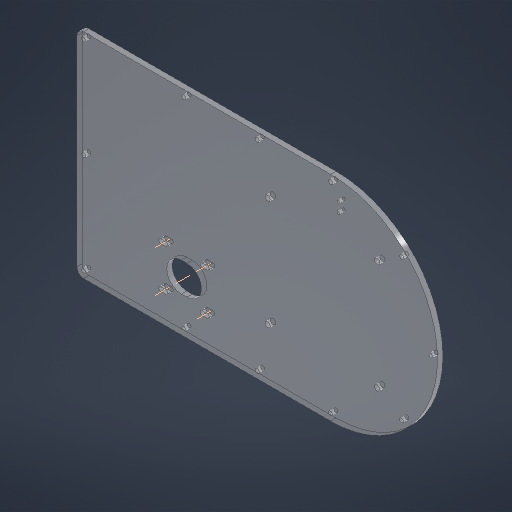
# Autodesk Inventor part: Base_solida
Saved by Autodesk Inventor 2025.2 (Build 292293000, 293)
## iProperties
Created: 2025-04-27
Part Number: Base_solida
Material: Generic
Document SubType Name: Modeling
Designer: Tiago
Density: 1 g/cm^3
Appearance: Polycarbonate - Clear
Mass: 159.889 g
Surface Area: 836.081 cm^2
Volume: 159.889 cm^3
Author: Tiago
Autodesk Inventor part; units mm, degrees
ref_plane "YZ Plane" through (0, 0, 0) normal (1, 0, 0) x (0, 1, 0)
ref_plane "XZ Plane" through (0, 0, 0) normal (0, 1, 0) x (-1, 0, 0)
ref_plane "XY Plane" through (0, 0, 0) normal (0, 0, 1) x (1, 0, 0)
sketch "Sketch1" plane through (0, 0, 0) normal (0, 0, 1) x (1, 0, 0)
  line L0 (-150, -80) -> (40, -80)
  line L1 (150, -80) -> (150, 80) construction
  line L2 (40, 80) -> (-150, 80)
  line L3 (-150, 80) -> (-150, -80)
  line L4 (-150, -80) -> (150, 80) construction
  line L5 (150, -80) -> (-150, 80) construction
  line L6 (-150, 0) -> (-107, 0) construction
  line L7 (-107, 0) -> (33.79, 0) construction
  line L8 (33.79, -41) -> (33.79, 41) construction
  line L9 (-7.21, 0) -> (74.79, 0) construction
  line L10 (33.79, 41) -> (74.79, 41) construction
  line L11 (74.79, 41) -> (74.79, 0) construction
  circle A0 centre (74.79, 41) radius 2
  circle A1 centre (74.79, -41) radius 2
  circle A2 centre (-7.21, 41) radius 2
  circle A3 centre (-7.21, -41) radius 2
  line L12 (33.79, 0) -> (33.79, 47) construction
  line L13 (33.79, 0) -> (33.79, -47) construction
  line L14 (-107, -80) -> (-107, -42.5) construction
  line L15 (-107, -42.5) -> (-77.5744, -42.5) construction
  line L16 (33.79, 0) -> (-69.7142, -42.5) construction
  circle A4 centre (-69.7142, -42.5) radius 11 construction
  line L17 (150, 0) -> (120, 0) construction
  line L18 (120, 0) -> (120, 0)
  arc A5 (40, -80) -> (120, 0) centre (40, 0) ccw
  arc A6 (120, 0) -> (40, 80) centre (40, 0) ccw
  line L19 (120, 0) -> (115, 0) construction
  circle A7 centre (115, 0) radius 1.5
  line L20 (40, 0) -> (111.7631, 71.7631) construction
  line L21 (96.5685, -56.5685) -> (93.033, -53.033) construction
  circle A8 centre (93.033, -53.033) radius 1.5
  line L22 (40, -80) -> (40, -75) construction
  circle A9 centre (40, -75) radius 1.5
  line L23 (40, -75) -> (-15, -75) construction
  line L24 (-15, -75) -> (-70, -75) construction
  line L25 (-150, -75) -> (-145, -75) construction
  circle A10 centre (-15, -75) radius 1.5
  circle A11 centre (-70, -75) radius 1.5
  circle A12 centre (-145, -75) radius 1.5
  circle A13 centre (-145, 0) radius 1.5
  circle A14 centre (93.033, 53.033) radius 1.5
  circle A15 centre (40, 75) radius 1.5
  circle A16 centre (-15, 75) radius 1.5
  circle A17 centre (-70, 75) radius 1.5
  circle A18 centre (-145, 75) radius 1.5
  line L26 (-145, -80) -> (-145, -75) construction
  line L27 (-150, 0) -> (-145, 0) construction
  line L28 (-71.7142, -42.5) -> (-67.7142, -42.5) construction
  line L29 (-85.2142, -42.5) -> (-54.2142, -42.5) construction
  line L30 (-69.7142, -27) -> (-69.7142, -58) construction
  line L31 (-69.7142, -27) -> (-85.2142, -27) construction
  line L32 (-85.2142, -27) -> (-85.2142, -42.5) construction
  circle A19 centre (-85.2142, -27) radius 1.5 construction
  circle A20 centre (-54.2142, -27) radius 1.5 construction
  circle A21 centre (-54.2142, -58) radius 1.5 construction
  circle A22 centre (-85.2142, -58) radius 1.5 construction
  line L33 (33.79, 0) -> (31.29, 0) construction
  line L34 (33.79, 0) -> (45.79, 0) construction
  line L35 (45.79, 0) -> (45.79, 58) construction
  circle A23 centre (45.79, 58) radius 1.1
  circle A24 centre (45.79, 65) radius 1.1
  line L36 (-83.2142, -27) -> (-87.2142, -27) construction
  arc A25 (-83.2142, -28.5) -> (-83.2142, -25.5) centre (-83.2142, -27) ccw
  line L37 (-83.2142, -28.5) -> (-87.2142, -28.5)
  line L38 (-83.2142, -25.5) -> (-87.2142, -25.5)
  arc A26 (-87.2142, -25.5) -> (-87.2142, -28.5) centre (-87.2142, -27) ccw
  circle A27 centre (-54.2142, -27) radius 1.5 construction
  line L39 (-56.2142, -27) -> (-52.2142, -27) construction
  arc A28 (-56.2142, -25.5) -> (-56.2142, -28.5) centre (-56.2142, -27) ccw
  line L40 (-56.2142, -28.5) -> (-52.2142, -28.5)
  line L41 (-56.2142, -25.5) -> (-52.2142, -25.5)
  arc A29 (-52.2142, -28.5) -> (-52.2142, -25.5) centre (-52.2142, -27) ccw
  line L42 (-69.7142, -58) -> (-85.2142, -58) construction
  circle A30 centre (-85.2142, -58) radius 1.5 construction
  circle A31 centre (-54.2142, -58) radius 1.5 construction
  line L43 (-83.2142, -58) -> (-87.2142, -58) construction
  arc A32 (-83.2142, -59.5) -> (-83.2142, -56.5) centre (-83.2142, -58) ccw
  line L44 (-83.2142, -56.5) -> (-87.2142, -56.5)
  line L45 (-83.2142, -59.5) -> (-87.2142, -59.5)
  arc A33 (-87.2142, -56.5) -> (-87.2142, -59.5) centre (-87.2142, -58) ccw
  line L46 (-56.2142, -56.5) -> (-52.2142, -56.5)
  arc A34 (-52.2142, -59.5) -> (-52.2142, -56.5) centre (-52.2142, -58) ccw
  line L47 (-56.2142, -58) -> (-52.2142, -58) construction
  circle A35 centre (-54.2142, -58) radius 1.5 construction
  line L48 (-56.2142, -59.5) -> (-52.2142, -59.5)
  arc A36 (-56.2142, -56.5) -> (-56.2142, -59.5) centre (-56.2142, -58) ccw
  arc A37 (-71.7142, -31.5) -> (-71.7142, -53.5) centre (-71.7142, -42.5) ccw
  arc A38 (-67.7142, -53.5) -> (-67.7142, -31.5) centre (-67.7142, -42.5) ccw
  arc A39 (-78.7016, -41.9742) -> (-78.7142, -42.5) centre (-67.7142, -42.5) ccw
  line L49 (-67.7142, -31.5) -> (-71.7142, -31.5)
  line L50 (-67.7142, -53.5) -> (-71.7142, -53.5)
  point P0 (0, 0)
  point P1 (120, -80)
  point P2 (120, 0)
  dimension "d0" = 300
  dimension "d1" = 160
  dimension "d4" = 43
  dimension "d6" = 140.79
  dimension "L_furos" = 82
  dimension "d9" = 82
  dimension "d11" = 4
  dimension "d30" = 47
  dimension "d40" = 37.5
  dimension "d45" = 111.89
  dimension "DN" = 22
  dimension "d47" = 30
  dimension "d49" = 80
  dimension "LF" = 5
  dimension "Furos" = 3
  dimension "d52" = 45
  dimension "d53" = 5
  dimension "d55" = 3
  dimension "d56" = 5
  dimension "d57" = 3
  dimension "d58" = 55
  dimension "d59" = 55
  dimension "d60" = 5
  dimension "d61" = 3
  dimension "d62" = 3
  dimension "d63" = 3
  dimension "d64" = 3
  dimension "d65" = 5
  dimension "d66" = 5
  dimension "d67" = 33.79
  dimension "d68" = 4
  dimension "d69" = 31
  dimension "d70" = 31
  dimension "FN" = 3
  dimension "d72" = 2.5
  dimension "d77" = 12
  dimension "NN" = 4
  dimension "d84" = 3
  dimension "d85" = 1.5
  dimension "d86" = 22
  dimension "d88" = 11
  dimension "d89" = 43
  dimension "d90" = 58
  dimension "d91" = 7
  dimension "d92" = 2.2
  dimension "d93" = 2.2
  constraints: 102 end point, 46 symmetric about line, 40 centre point, 35 coincident, 27 point on circle, 13 horizontal, 12 tangent, 11 midpoint, 10 point on line, 7 perpendicular, 5 vertical, 2 parallel, 2 vertical alignment, 1 concentric, 21 other
  measures "d0" distance of L2.end L1.end
  measures "d1" distance of L1.start L1.end
  measures "d4" distance of L6.start L6.end
  measures "d6" distance of L7.start L7.end
  measures "L_furos" distance of L8.start L8.end
  measures "d9" distance of L9.start L9.end
  measures "d11" diameter of A0
  measures "d30" distance of L12.start L12.end
  measures "d40" distance of L14.start L14.end
  measures "d45" distance of L12.start L16.end
  measures "DN" diameter of A4
  measures "d47" distance of L17.start L17.end
  measures "d49" radius of A5
  measures "LF" distance of L18.end L19.end
  measures "Furos" diameter of A7
  measures "d52" angle of L9 L20
  measures "d53" distance of L21.start L21.end
  measures "d55" diameter of A8
  measures "d56" distance of L0.end L22.end
  measures "d57" diameter of A9
  measures "d58" distance of L23.start L23.end
  measures "d59" distance of L23.end L24.end
  measures "d60" distance of L25.end L25.start
  measures "d61" diameter of A10
  measures "d62" diameter of A11
  measures "d63" diameter of A12
  measures "d64" diameter of A13
  measures "d65" distance of L26.start L25.end
  measures "d66" distance of L6.start L27.end
  measures "d67" distance of L7.end point (0, 0)
  measures "d68" distance of L28.start L28.end
  measures "d69" distance of L29.start L29.end
  measures "d70" distance of L30.start L30.end
  measures "FN" diameter of A19
  measures "d72" distance of L33.start L33.end
  measures "d77" distance of L33.start L34.end
  measures "NN" distance of L36.start L36.end
  measures "d84" diameter of A25
  measures "d85" radius of A26
  measures "d86" diameter of A37
  measures "d88" radius of A38
  measures "d89" distance of L0.start L14.start
  measures "d90" distance of L34.end L35.end
  measures "d91" distance of A24.centre L35.end
  measures "d92" diameter of A23
  measures "d93" diameter of A24
extrude "Extrusion1" add sketch "Sketch1" along normal blind 4 contours L3 L2 A6 A5 L0 | A23 | A24
extrude "Extrusion5" cut sketch "Sketch1" along normal up to surface (4 mm away) contours A23 | A24
fillet "Fillet1" radius 5 2 edges at (-150, -80, 2) (-150, 80, 2)
equation "\"d9\" = L_furos"
equation "\"d53\" = LF"
equation "\"d55\" = Furos"
equation "\"d56\" = LF"
equation "\"d57\" = Furos"
equation "\"d60\" = LF"
equation "\"d61\" = Furos"
equation "\"d62\" = Furos"
equation "\"d63\" = Furos"
equation "\"d64\" = Furos"
equation "\"d65\" = LF"
equation "\"d66\" = LF"
body "Solid1"
